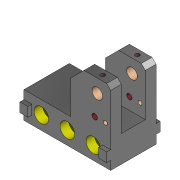
# Autodesk Inventor part: TL20240701-10200AT-001
Saved by Autodesk Inventor 2022.5 (Build 265521000, 521)
## iProperties
Category: ANTI BACK ASSY
Company: 현대트랜시스(대유)
RuleStatus: InUse
Part Number: TL20240701-10200AT-001
Project: SW-PJT
Checked By: 김형민
Engr Approved By: 김시현
User Status: 1 x13
Material: AL6061
Description: 0
Document SubType Name: Modeling
Mfg Approved By: 호상태
Designer: USER106
Stock Number: 001
Density: 2.7 g/cm^3
Appearance: Anodizing White
Detail Description: Processed products
Title: BASE BLOCK
Subject: SW차종 시트조립라인
Author: USER106
Revision Number: A
Autodesk Inventor part; units mm, degrees
ref_plane "YZ Plane" through (0, 0, 0) normal (1, 0, 0) x (0, 1, 0)
ref_plane "XZ Plane" through (0, 0, 0) normal (0, 1, 0) x (-1, 0, 0)
ref_plane "XY Plane" through (0, 0, 0) normal (0, 0, 1) x (1, 0, 0)
sketch "Sketch2" plane through (0, 0, 0) normal (1, 0, 0) x (0, 1, 0)
  line L0 (17, -27.5) -> (-17, -27.5)
  line L1 (-17, -27.5) -> (-17, 27.5)
  line L2 (-17, 27.5) -> (17, 27.5)
  line L3 (17, 27.5) -> (17, -27.5)
  line L4 (17, -27.5) -> (-17, 27.5) construction
  line L5 (-17, -27.5) -> (17, 27.5) construction
  line L6 (9, 27.5) -> (-9, 27.5)
  line L7 (-9, 27.5) -> (-9, -7.5)
  line L8 (-9, -7.5) -> (9, -7.5)
  line L9 (9, -7.5) -> (9, 27.5)
  point P0 (0, 0)
  point P1 (-9, 27.5)
  dimension "d1" = 34
  dimension "d2" = 55
  dimension "d3" = 8
  dimension "d4" = 8
  dimension "d5" = 20
  constraints: 20 end point, 4 parallel, 2 horizontal, 2 midpoint, 2 perpendicular, 1 point on line
  measures "d1" distance of L1.end L2.end
  measures "d2" distance of L0.end L1.end
  measures "d3" distance between parallel lines of L1 L7
  measures "d4" distance between parallel lines of L3 L9
  measures "d5" distance between parallel lines of L8 L0
extrude "Extrusion1" add sketch "Sketch2" along normal mid plane 65 contours L0 L1 L2 L7 L8 L9 L3
sketch "Sketch3" plane through (0, 0, 0) normal (0, 1, 0) x (-1, 0, 0)
  line L0 (32.5, 27.5) -> (-32.5, 27.5) projected
  line L1 (32.5, 27.5) -> (-2.5, 27.5)
  line L2 (-2.5, 27.5) -> (-2.5, -7.5)
  line L3 (-2.5, -7.5) -> (32.5, -7.5)
  line L4 (32.5, -7.5) -> (32.5, 27.5)
  point P0 (0, 0)
  dimension "d8" = 35
  dimension "d9" = 35
  constraints: 8 end point, 2 parallel, 1 horizontal, 1 perpendicular
  measures "d8" distance of L3.end L2.end
  measures "d9" distance of L2.end L1.end
extrude "Extrusion2" cut sketch "Sketch3" along normal through all both and the other way through all
sketch "Sketch4" plane through (32.5, 0, 0) normal (1, 0, 0) x (0, 0, -1)
  line L0 (21, -17) -> (14, -17)
  line L1 (14, -17) -> (14, -20)
  line L2 (14, -20) -> (21, -20)
  line L3 (21, -20) -> (21, -17)
  line L4 (27.5, -17) -> (27.5, 17) projected
  line L5 (-27.5, -17) -> (27.5, -17) projected
  line L6 (27.5, 17) -> (27.5, -17) projected
  line L7 (27.5, 0) -> (7.5, 0) construction
  line L8 (7.5, -17) -> (7.5, 17) projected
  line L9 (21, 17) -> (14, 17)
  line L10 (14, 17) -> (14, 20)
  line L11 (14, 20) -> (21, 20)
  line L12 (21, 20) -> (21, 17)
  point P0 (0, 0)
  dimension "d12" = 7
  dimension "d13" = 3
  dimension "d14" = 6.5
  constraints: 18 end point, 4 symmetric about line, 2 midpoint, 2 parallel, 1 horizontal, 1 perpendicular, 1 point on line
  measures "d12" distance of L2.end L1.end
  measures "d13" distance of L1.end L0.end
  measures "d14" distance between parallel lines of L3 L4
extrude "Extrusion3" add sketch "Sketch4" against normal blind 6
extrude "Extrusion4" add sketch "Sketch4" along normal blind 6 from surface at -65
sketch "Sketch5" plane through (-32.5, -17, -27.5) normal (0, -1, 0) x (1, 0, 0)
  line L0 (65, 0) -> (0, 0) projected
  line L1 (65, 6.5) -> (65, 0) projected
  point P0 (32.5, 27.5)
  point P1 (13, 10)
  point P2 (32.5, 10)
  point P3 (52, 10)
  dimension "d19" = 10
  dimension "d20" = 13
  dimension "d21" = 19.5
  dimension "d22" = 19.5
  constraints: 2 horizontal alignment
  measures "d19" distance from line of point (52, 10) L0
  measures "d20" distance from line of point (52, 10) L1
  measures "d21" distance of point (32.5, 10) point (52, 10)
  measures "d22" distance of point (13, 10) point (32.5, 10)
hole "Hole1" at (-19.5, -17, -17.5) at (0, -17, -17.5) at (19.5, -17, -17.5) direction (0, 1, 0) diameter 6.6 end through all counterbore diameter 11 counterbore depth 6.5 clearance for "Socket Head Cap Screw" size "M6" standard "TS Profile"
sketch "Sketch6" plane through (-32.5, 17, -27.5) normal (0, 1, 0) x (1, 0, 0)
  circle A0 centre (52, -10) radius 3.3 projected
  circle A1 centre (32.5, -10) radius 3.3 projected
  circle A2 centre (13, -10) radius 3.3 projected
  point P0 (32.5, -27.5)
  constraints: 3 coincident
hole "Hole2" at (19.5, 17, -17.5) at (0, 17, -17.5) at (-19.5, 17, -17.5) direction (0, -1, 0) diameter 6.6 end through all counterbore diameter 11 counterbore depth 6.5 clearance for "Socket Head Cap Screw" size "M6" standard "TS Profile"
sketch "Sketch7" plane through (-32.5, -17, -27.5) normal (0, -1, 0) x (1, 0, 0)
  line L0 (65, 0) -> (0, 0) projected
  line L1 (65, 55) -> (65, 13.5) projected
  point P0 (32.5, 27.5)
  point P1 (61, 29)
  dimension "d37" = 29
  dimension "d38" = 4
  measures "d37" distance from line of point (61, 29) L0
  measures "d38" distance from line of L1 point (61, 29)
hole "Hole3" at (28.5, -17, 1.5) direction (0, 1, 0) diameter 3 end through all
sketch "Sketch8" plane through (-32.5, -17, -27.5) normal (0, -1, 0) x (1, 0, 0)
  line L0 (35, 55) -> (65, 55) projected
  line L1 (65, 55) -> (65, 13.5) projected
  point P0 (32.5, 27.5)
  point P1 (55, 45)
  dimension "d46" = 10
  dimension "d47" = 10
  measures "d46" distance from line of point (55, 45) L0
  measures "d47" distance from line of point (55, 45) L1
hole "Hole4" at (22.5, -17, 17.5) direction (0, 1, 0) diameter 8 end through all
sketch "Sketch9" plane through (32.5, -17, 27.5) normal (0, 0, 1) x (1, 0, 0)
  line L0 (-30, 34) -> (0, 34) projected
  line L1 (-30, 0) -> (0, 0) projected
  line L2 (0, 8) -> (0, 0) projected
  point P0 (-32.5, 17)
  point P1 (-10, 4)
  point P2 (-10, 30)
  dimension "d55" = 4
  dimension "d56" = 4
  dimension "d57" = 10
  constraints: 1 vertical alignment
  measures "d55" distance from line of point (-10, 30) L0
  measures "d56" distance from line of point (-10, 4) L1
  measures "d57" distance from line of point (-10, 4) L2
hole "Hole5" at (22.5, -13, 27.5) at (22.5, 13, 27.5) direction (0, 0, -1) diameter 3.242 depth 10 tip angle 118 thread size "M4x0.7" class "6H" standard "TS profile"
chamfer "Chamfer1" distance 10 angle 45 2 edges at (2.5, -13, 27.5) (2.5, 13, 27.5)
chamfer "Chamfer2" distance 3 angle 45 2 edges at (32.5, -13, 27.5) (32.5, 13, 27.5)
sketch "Sketch10" plane through (-32.5, 17, -27.5) normal (0, 1, 0) x (1, 0, 0)
  circle A0 centre (53, -29) radius 2.5 construction
  line L0 (0, 0) -> (65, 0) projected
  line L1 (65, 0) -> (65, -6.5) projected
  dimension "d71" = 5
  dimension "d72" = 29
  dimension "d74" = 12
  constraints: 1 centre point
  measures "d71" diameter of A0
  measures "d72" distance from line of A0.centre L0
  measures "d74" distance from line of L1 A0.centre
hole "Hole6" at (20.5, 17, 1.5) direction (0, -1, 0) diameter 4.134 end through all thread size "M5x0.8" class "6H" standard "TS profile"
equation "\"d56\" = d55"
body "Solid1"
